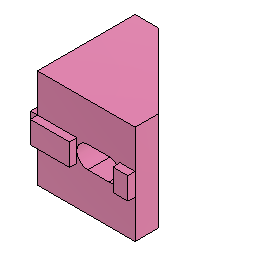
simplified_backet_for_print v2 (Autodesk Fusion 360 design; units mm, degrees)
Autodesk Fusion 360 part; units mm, degrees
note: some values were not read from the file. Set by a fixed rule: which face or edge a step refers to.
sketch "Sketch1" plane through (0, 0, 0) normal (0, 0, 1) x (1, 0, 0)
  line L0 (0, 0) -> (41.23, 0)
  line L1 (41.23, 0) -> (41.23, 41.23)
  line L2 (41.23, 41.23) -> (0, 41.23)
  line L3 (0, 41.23) -> (0, 0)
  line L4 (0, 0) -> (41.23, 41.23) construction
  line L5 (9.8, 41.23) -> (41.23, 9.8)
  dimension "d1" = 41.23
  dimension "d2" = 41.23
  dimension "d3" = 9.8
  constraint horizontal L0
  constraint vertical L1
  constraint horizontal L2
  constraint vertical L3
  constraint coincident L0.start L3.end
  constraint coincident L2 L5.start
  constraint coincident L1 L5.end
  constraint perpendicular L4 L5
  measures "d1" distance of L0.start L0.end
  measures "d2" distance of L0.start L2.end
  measures "d3" distance of L2.end L5.start
extrude "Extrude1" add sketch "Sketch1" along normal mid plane 41.8 contours L0 L1 L2 L3 L5
shell "Shell1" thickness 3.4 removed faces 3 at (6.5333, 41.23, 6.9667) at (30.7533, 20.2767, 6.9667) at (41.23, 3.2667, 6.9667)
move_face "OffsetFaces1" offset 6.4 1 faces at (16.01, 3.4, 5.8333)
move_face "OffsetFaces2" offset 6.4 1 faces at (3.4, 30.7533, -5.8333)
sketch "Sketch2" plane through (9.8, 0, 0) normal (1, 0, 0) x (0, 1, 0)
  line L0 (9.8, 17.5) -> (9.8, -17.5)
  line L1 (9.8, -17.5) -> (41.23, -17.5)
  line L2 (41.23, -17.5) -> (41.23, 17.5)
  line L3 (41.23, 17.5) -> (9.8, 17.5)
  line L4 (0, 0) -> (41.23, 0) construction
  line L5 (21.28, -4.65) -> (30.18, -4.65)
  arc A0 (30.18, -4.65) -> (30.18, 4.65) centre (30.18, 0) ccw
  line L6 (30.18, 4.65) -> (21.28, 4.65)
  arc A1 (21.28, 4.65) -> (21.28, -4.65) centre (21.28, 0) ccw
  line L7 (21.28, 0) -> (30.18, 0) construction
  line L8 (30.18, 0) -> (34.83, 0) construction
  line L9 (21.28, 0) -> (16.63, 0) construction
  dimension "d9" = 6.4
  dimension "d10" = 18.2
  dimension "d11" = 9.3
  constraint coincident L4.start origin
  constraint midpoint L2 L4.end
  constraint tangent L5 A0
  constraint tangent A0 L6
  constraint parallel L5 L6
  constraint tangent L6 A1
  constraint tangent L5 A1
  constraint coincident L4 A0.centre
  constraint parallel L4 L7
  constraint coincident A0.centre L7.end
  constraint midpoint A0 L8.end
  constraint coincident A1.centre L7.start
  constraint midpoint A1 L9.end
  measures "d9" distance of L4.end L8.end
  measures "d10" distance of L8.end L9.end
  measures "d11" distance of L5 L6
extrude "Extrude2" cut sketch "Sketch2" against normal through all contours L5 A0 L6 A1
sketch "Sketch4" plane through (0, 0, 0) normal (-1, 0, 0) x (0, -1, 0)
  line L0 (-30.18, 4.65) -> (-21.28, 4.65)
  arc A0 (-21.28, -4.65) -> (-21.28, 4.65) centre (-21.28, 0) ccw
  line L1 (-21.28, -4.65) -> (-30.18, -4.65)
  arc A1 (-30.18, 4.65) -> (-30.18, -4.65) centre (-30.18, 0) ccw
  line L2 (0, -20.9) -> (0, 20.9)
  line L3 (0, 20.9) -> (-41.23, 20.9)
  line L4 (-41.23, 20.9) -> (-41.23, -20.9)
  line L5 (-41.23, -20.9) -> (0, -20.9)
  line L6 (-41.23, 4.75) -> (0, 4.75)
  line L7 (0, 4.75) -> (0, -4.75)
  line L8 (0, -4.75) -> (-41.23, -4.75)
  line L9 (-41.23, -4.75) -> (-41.23, 4.75)
  line L10 (-41.23, 4.75) -> (0, -4.75) construction
  line L11 (0, 4.75) -> (-41.23, -4.75) construction
  line L12 (0, 0) -> (-20.615, 0) construction
  arc A2 (-30.18, 4.65) -> (-30.18, -4.65) centre (-30.18, 0) ccw
  arc A3 (-21.28, -4.65) -> (-21.28, 4.65) centre (-21.28, 0) ccw
  line L13 (-34.63, 4.75) -> (-25.73, 4.75)
  line L14 (-25.73, 4.75) -> (-25.73, -4.75) construction
  line L15 (-25.73, -4.75) -> (-34.63, -4.75)
  line L16 (-34.63, 4.75) -> (-25.73, -4.75) construction
  line L17 (-25.73, 4.75) -> (-34.63, -4.75) construction
  line L18 (-34.83, 4.75) -> (-16.63, 4.75)
  line L19 (-16.63, 4.75) -> (-16.63, -4.75)
  line L20 (-16.63, -4.75) -> (-34.83, -4.75)
  line L21 (-34.83, -4.75) -> (-34.83, 4.75)
  line L22 (-34.83, 4.75) -> (-16.63, -4.75) construction
  line L23 (-16.63, 4.75) -> (-34.83, -4.75) construction
  point P0 (-20.615, 0)
  point P1 (-30.18, 0)
  point P2 (-25.73, 0)
  dimension "d28" = 9.5
  constraint horizontal L6
  constraint perpendicular L6 L7
  constraint parallel L6 L8
  constraint parallel L7 L9
  constraint coincident L10 P0
  constraint coincident L11 P0
  constraint coincident L4 L6.start
  constraint coincident L2 L6.end
  constraint coincident L12.start origin
  constraint coincident P0 L12.end
  constraint horizontal L12
  constraint horizontal L13
  constraint perpendicular L13 L14
  constraint parallel L13 L15
  constraint coincident L16 P1
  constraint coincident L17 P1
  constraint coincident L6 L13.start
  constraint coincident P1 A1.centre
  constraint horizontal L18
  constraint perpendicular L18 L19
  constraint parallel L18 L20
  constraint parallel L19 L21
  constraint coincident L22 P2
  constraint coincident L23 P2
  constraint coincident L6 L18.start
  constraint midpoint L14 P2
  constraint tangent A1 L21
  constraint tangent A0 L19
  measures "d28" distance of L6 L8
extrude "Extrude5" add sketch "Sketch4" along normal blind 3 draft -2 contours L4 L6 L8 L9 L21 | L2 L6 L7 L8 L19
ref_plane "WorkPlane3" through (0, 0, -12.825) normal (-0.707107, 0.707107, 0) x (0, 0, 1)
mirror "Mirror3" about plane through (0, 0, -12.825) normal (-0.707107, 0.707107, 0) of "Extrude2", "Extrude5"
